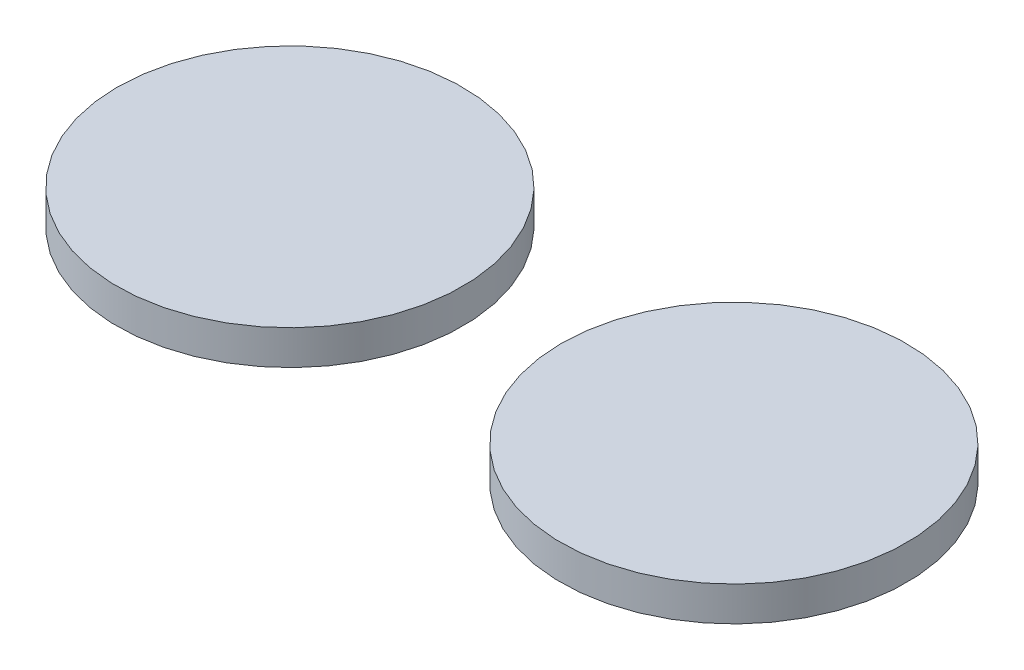
# Autodesk Inventor part: foundation dummy
Saved by Autodesk Inventor 2025.1 (Build 291241020, 241B)
## iProperties
Created: 2025-01-24
Part Number: foundation dummy
Material: Generic
Document SubType Name: Modeling
Designer: user
Density: 1 g/cm^3
Appearance: Default
Author: user
Autodesk Inventor part; units mm, degrees
ref_plane "YZ Plane" through (0, 0, 0) normal (1, 0, 0) x (0, 1, 0)
ref_plane "XZ Plane" through (0, 0, 0) normal (0, 1, 0) x (-1, 0, 0)
ref_plane "XY Plane" through (0, 0, 0) normal (0, 0, 1) x (1, 0, 0)
sketch "Sketch1" plane through (0, 0, 0) normal (0, 1, 0) x (-1, 0, 0)
  circle A0 centre (-900, 0) radius 700
  circle A1 centre (900, 0) radius 700
  line L0 (0, 0) -> (0, 700) construction
  line L1 (-200, 0) -> (-200, 700) construction
  line L2 (200, 0) -> (200, 700) construction
  line L3 (-900, 0) -> (-900, 700) construction
  line L4 (1600, 0) -> (-1600, 0) construction
  dimension "d0" = 400
  dimension "d1" = 1400
  dimension "d5" = 3200
  constraints: 10 end point, 5 point on circle, 4 vertical, 2 centre point, 2 horizontal alignment, 2 parallel, 2 tangent, 1 coincident, 1 horizontal, 1 midpoint, 1 other
  measures "d0" distance between parallel lines of L2 L1
  measures "d1" diameter of A0
  measures "d5" distance of L4.start L4.end
extrude "Extrusion1" add sketch "Sketch1" against normal blind 140
body "Solid1"
